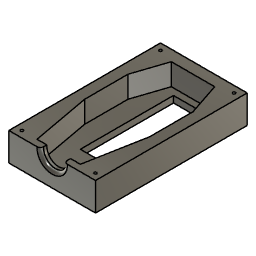
NEMA 14 50 Window mount (Autodesk Fusion 360 design; units mm, degrees)
part number: 2025-06-09-03-43-27-146
Autodesk Fusion 360 part; units mm, degrees
cylinder "CylinderPrimitive1" add diameter 54.864 height 97.155 placed x (1, 0, 0) y (0, 1, 0) z (0, 0, 1) at (0, 0, 0) makes body 1
cylinder "CylinderPrimitive2" add diameter 45.085 height 101.6 placed x (1, 0, 0) y (0, 0, -1) z (0, 1, 0) at (0, 0, 0) separate body makes body 2
move_body "Move1" bodies 2 to x (1, 0, 0) y (0, 1, 0) z (0, 0, 1) at (0, -74.168, 74.93)
move_body "Move2" bodies 2 to x (1, 0, 0) y (0, 1, 0) z (0, 0, 1) at (0, 0, -20.32)
move_face "OffsetFaces1" offset -53.34 1 faces at (4.8978, 1.8188, 0) on bodies 1
box "BoxPrimitive1" add length 101.6 width 25.4 height 40.64 placed x (0, -1, 0) y (1, 0, 0) z (0, 0, 1) at (-12.7, 27.432, 0) separate body makes body 3
sketch "Sketch4" plane through (0, 0, 0) normal (0, 0, 1) x (1, 0, 0)
  spline S0 degree 2 poles (-33.02, -12.7) (0, 12.7) (33.02, -12.7) knots 0 0 0 7.015668 7.015668 7.015668 weights 1 0.873063 1
  line L0 (33.02, -12.7) -> (33.02, -38.1)
  line L1 (33.02, -38.1) -> (26.67, -50.8)
  line L2 (26.67, -50.8) -> (20.32, -88.9)
  line L3 (20.32, -88.9) -> (-20.32, -88.9)
  line L4 (-20.32, -88.9) -> (-26.67, -50.8)
  line L5 (-26.67, -50.8) -> (-33.02, -38.1)
  line L6 (-33.02, -38.1) -> (-33.02, -12.7)
  constraint vertical L0
  constraint horizontal L3
  constraint vertical L6
extrude "Extrude1" add sketch "Sketch4" along normal blind 7.62 separate body makes body 4
move_body "Move3" bodies 4 to x (1, 0, 0) y (0, 1, 0) z (0, 0, 1) at (0, 0, 50.8)
fillet "Fillet1" radius 2.54 8 edges at (33.02, -12.7, 54.61) (33.02, -38.1, 54.61) (26.67, -50.8, 54.61) (20.32, -88.9, 54.61) (-33.02, -12.7, 54.61) (-33.02, -38.1, 54.61) (-26.67, -50.8, 54.61) (-20.32, -88.9, 54.61) on bodies 4
move_body "Move4" bodies 4 to x (1, 0, 0) y (0, 1, 0) z (0, 0, 1) at (0, 5.08, 0)
fillet "Fillet2" radius 12.7 2 edges at (0, 27.432, 0) (0, -74.168, 0) on bodies 3
combine "Combine1" operation add target body 1 tool bodies 2 3 4
box "BoxPrimitive2" add length 177.8 width 101.6 height 33.02 placed x (0, -1, 0) y (1, 0, 0) z (0, 0, 1) at (-50.8, 38.1, 0) separate body makes body 5
move_body "Move5" bodies 5 to x (1, 0, 0) y (0, 1, 0) z (0, 0, 1) at (0, 0, 55.88)
move_body "Move6" bodies 5 to x (1, 0, 0) y (0, 1, 0) z (0, 0, 1) at (0, 12.7, 0)
copy_body "CopyPasteBodies1" bodies 5 makes body 6
move_body "Move7" bodies 6 to x (1, 0, 0) y (0, 1, 0) z (0, 0, 1) at (0, 0, -33.02)
cylinder "CylinderPrimitive3" cut diameter 56.388 height -33.02 placed x (1, 0, 0) y (0, 1, 0) z (0, 0, 1) at (0, 0, 88.9) bodies 5
sketch "Sketch9" plane through (0, 0, 55.88) normal (0, 0, -1) x (1, 0, 0)
  circle A0 centre (0, 0) radius 28.194
  line L0 (50.8, 127) -> (-50.8, 127)
  line L1 (-50.8, 127) -> (-50.8, -50.8)
  line L2 (-50.8, -50.8) -> (50.8, -50.8)
  line L3 (50.8, -50.8) -> (50.8, 127)
  line L4 (25.4, 119.38) -> (-25.4, 119.38)
  line L5 (-25.4, 119.38) -> (-38.1, 50.8)
  line L6 (-38.1, 50.8) -> (-38.1, 0)
  line L7 (-38.1, 0) -> (-25.4, -38.1)
  line L8 (-25.4, -38.1) -> (25.4, -38.1)
  line L9 (25.4, -38.1) -> (38.1, 0)
  line L10 (38.1, 0) -> (38.1, 50.8)
  line L11 (38.1, 50.8) -> (25.4, 119.38)
  constraint perpendicular L3 L4
  constraint perpendicular L4 L6
  constraint perpendicular L6 L8
  constraint perpendicular L2 L10
extrude "Extrude2" cut sketch "Sketch9" against normal blind 22.86 contours L4 L5 L6 L7 L8 L9 L10 L11 bodies 5
extrude "Extrude3" cut sketch "Sketch9" along normal blind 25.4 contours L4 L5 L6 L7 L8 L9 L10 L11 bodies 6
box "BoxPrimitive3" cut length 109.22 width 30.48 height -7.62 placed x (0, 1, 0) y (1, 0, 0) z (0, 0, -1) at (-15.24, -78.74, 22.86) bodies 6
cylinder "CylinderPrimitive4" cut diameter 27.94 height 76.2 placed x (1, 0, 0) y (0, 0, 1) z (0, -1, 0) at (0, -74.168, 54.61) bodies 5 6
fillet "Fillet3" radius 3.81 2 edges at (0, -127, 68.58) (0, -127, 40.64) on bodies 5 6
sketch "Sketch12" plane through (0, 0, 22.86) normal (0, 0, -1) x (1, 0, 0)
  line L0 (-15.24, -30.48) -> (-15.24, 78.74)
  line L1 (-15.24, 78.74) -> (15.24, 78.74)
  line L2 (15.24, 78.74) -> (15.24, -30.48)
  line L3 (15.24, -30.48) -> (-15.24, -30.48)
  line L4 (50.8, 127) -> (-50.8, 127)
  line L5 (-50.8, 127) -> (-50.8, -50.8)
  line L6 (-50.8, -50.8) -> (50.8, -50.8)
  line L7 (50.8, -50.8) -> (50.8, 127)
  circle A0 centre (43.18, -43.18) radius 1.6002
  circle A1 centre (-43.18, -43.18) radius 1.6002
  circle A2 centre (43.18, 119.38) radius 1.6002
  circle A3 centre (-43.18, 119.38) radius 1.6002
  dimension "d42" = 3.2004
  dimension "d43" = 3.2004
  dimension "d44" = 3.2004
  dimension "d45" = 3.2004
  measures "d42" diameter of A0
  measures "d43" diameter of A1
  measures "d44" diameter of A2
  measures "d45" diameter of A3
extrude "Extrude4" cut sketch "Sketch12" against normal blind 58.42 contours A0 | A1 | A2 | A3 bodies 5 6
sketch "Sketch13" plane through (0, 0, 22.86) normal (0, 0, -1) x (1, 0, 0)
  circle A0 centre (-43.18, 119.38) radius 1.6002
  circle A1 centre (-43.18, -43.18) radius 1.6002
  circle A2 centre (43.18, 119.38) radius 1.6002
  circle A3 centre (43.18, -43.18) radius 1.6002
  line L0 (-15.24, -30.48) -> (-15.24, 78.74)
  line L1 (-15.24, 78.74) -> (15.24, 78.74)
  line L2 (15.24, 78.74) -> (15.24, -30.48)
  line L3 (15.24, -30.48) -> (-15.24, -30.48)
  line L4 (50.8, 127) -> (-50.8, 127)
  line L5 (-50.8, 127) -> (-50.8, -50.8)
  line L6 (-50.8, -50.8) -> (50.8, -50.8)
  line L7 (50.8, -50.8) -> (50.8, 127)
  circle A4 centre (43.18, -43.18) radius 3
  circle A5 centre (-43.18, -43.18) radius 3
  circle A6 centre (-43.18, 119.38) radius 3
  circle A7 centre (43.18, 119.38) radius 3
  dimension "d48" = 6
  dimension "d49" = 6
  dimension "d50" = 6
  dimension "d51" = 6
  constraint concentric A3 A4
  constraint concentric A1 A5
  constraint concentric A0 A6
  constraint concentric A2 A7
  measures "d48" diameter of A4
  measures "d49" diameter of A5
  measures "d50" diameter of A6
  measures "d51" diameter of A7
extrude "Extrude5" cut sketch "Sketch13" against normal blind 7.62 contours A4 | A5 | A6 | A7 bodies 6
move_face "OffsetFaces2" offset -25.4 1 faces at (4.699, -8.1389, 55.88) on bodies 6
hidden bodies 1 5
named bodies: "Plug", "Front Face plate", "Rear plate"
